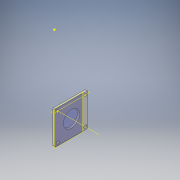
# Autodesk Inventor part: 30_Adapterplate_Eyepiece
Saved by Autodesk Inventor 2019 (Build 230136000, 136)
## iProperties
Created: 2018-06-14
Part Number: 30_Adapterplate_Eyepiece
Material: Generisch
Document SubType Name: Modeling
Designer: diederichbenedict
Density: 1 g/cm^3
Appearance: Vorgabe
Author: diederichbenedict
Autodesk Inventor part; units mm, degrees
ref_plane "YZ Plane" through (0, 0, 0) normal (1, 0, 0) x (0, 1, 0)
ref_plane "XZ Plane" through (0, 0, 0) normal (0, 1, 0) x (-1, 0, 0)
ref_plane "XY Plane" through (0, 0, 0) normal (0, 0, 1) x (1, 0, 0)
ref_plane "Arbeitsebene1" through (0, 0, -149.8) normal (-1, 0, 0) x (0, 0, 1)
sketch "Skizze1" plane through (0, 0, -149.8) normal (-1, 0, 0) x (0, 0, 1)
  circle A0 centre (44.9, 5) radius 1.5 construction
  circle A1 centre (4.9, 5) radius 1.5 construction
  circle A2 centre (4.9, 45) radius 1.6 construction
  circle A3 centre (44.9, 45) radius 1.6 construction
  line L0 (39.5269, 16.1776) -> (39.5269, 39.7) construction
  line L1 (16.0815, 10.3) -> (33.7185, 10.3) construction
  line L2 (10.2731, 16.1776) -> (10.2731, 39.7) construction
  circle A4 centre (24.9, 24.9269) radius 14.6269 construction
  line L3 (2, 49.8269) -> (47.8, 49.8269)
  line L4 (49.8, 47.8269) -> (49.8, 2.0269)
  line L5 (47.8, 0.0269) -> (2, 0.0269)
  line L6 (0, 2.0269) -> (0, 47.8269)
  line L7 (0, 49.8269) -> (49.8, 0.0269) construction
  line L8 (49.8, 49.8269) -> (0, 0.0269) construction
  arc A5 (47.8, 0.0269) -> (49.8, 2.0269) centre (47.8, 2.0269) ccw
  arc A6 (0, 2.0269) -> (2, 0.0269) centre (2, 2.0269) ccw
  arc A7 (2, 49.8269) -> (0, 47.8269) centre (2, 47.8269) ccw
  arc A8 (49.8, 47.8269) -> (47.8, 49.8269) centre (47.8, 47.8269) ccw
  line L9 (2, 1.0269) -> (47.8, 1.0269)
  arc A9 (47.8, 1.0269) -> (48.8, 2.0269) centre (47.8, 2.0269) ccw
  line L10 (48.8, 2.0269) -> (48.8, 47.8269)
  arc A10 (48.8, 47.8269) -> (47.8, 48.8269) centre (47.8, 47.8269) ccw
  line L11 (47.8, 48.8269) -> (2, 48.8269)
  arc A11 (2, 48.8269) -> (1, 47.8269) centre (2, 47.8269) ccw
  line L12 (1, 47.8269) -> (1, 2.0269)
  arc A12 (1, 2.0269) -> (2, 1.0269) centre (2, 2.0269) ccw
  point P0 (149.8, 0)
extrude "Extrusion1" add sketch "Skizze1" along normal blind 3 contours A12 L12 A11 L11 A10 L10 A9 L9
ref_plane "Arbeitsebene2" through (0, 5, -104.9) normal (0, 0, 1) x (1, 0, 0)
sketch "Skizze2" plane through (0, 5, -104.9) normal (0, 0, 1) x (1, 0, 0)
  line L0 (0, 5.3) -> (7, 5.3) projected
  line L1 (0, 8.3139) -> (7.3731, 8.3139)
  line L2 (0, -2.9731) -> (0, 42.8269) projected
  line L3 (0, 6.807) -> (-3, 6.807)
  line L4 (-3, -2.9731) -> (-3, 42.8269) projected
  circle A0 centre (-1.5, 6.807) radius 2.6
  line L5 (1.1, 6.807) -> (-4.1, 6.807)
  line L6 (0, 1.6861) -> (7.3731, 1.6861)
  line L7 (2.4, -2.5) -> (8, -2.5) projected
  line L8 (15, -1.5) -> (6.4, -1.5)
  line L9 (10.2731, 1.5) -> (6.4, 1.5)
  line L10 (0, -0.0077) -> (-3, -0.0077)
  circle A1 centre (-1.5, -0.0077) radius 2.6
  line L11 (1.1, -0.0077) -> (-4.1, -0.0077)
  line L12 (-7.92, 0) -> (18.82, 0) projected
  point P0 (0, -5)
  point P1 (0, 1.4993)
  dimension "d6" = 1.507
  dimension "d7" = 5.2
  dimension "d9" = 5.2
  constraints: 16 end point, 8 horizontal, 4 point on circle, 2 centre point, 2 midpoint, 2 point on line, 9 other
  measures "d6" distance between parallel lines of L0 L3
  measures "d7" diameter of A0
  measures "d9" diameter of A1
revolve "Umdrehung2" cut sketch "Skizze2" angle 360 about axis through (47.3, 5, -104.9) along (1, 0, 0) contours L11 A1 L2 | L2 A1 L4 L10 | L4 A1 L11
pattern_linear "Rechteckige Anordnung1" count 2 spacing 40 along (0, 1, 0) count 2 spacing 40 along (0, 0, -1) of "Umdrehung2"
sketch "Skizze3" plane through (0, 0, -149.8) normal (1, 0, 0) x (0, 0, -1)
  point P0 (-149.8, 0)
sketch "Skizze4" plane through (0, 0, -149.8) normal (1, 0, 0) x (0, 0, -1)
  circle A0 centre (-24.9, 25) radius 11.45
  circle A1 centre (-24.9, 25) radius 11.75
  point P0 (-149.8, 0)
  dimension "d18" = 0.3
  constraints: 2 centre point, 2 other
  measures "d18" radial gap between concentric circles of A0 A1
extrude "Extrusion2" cut sketch "Skizze4" against normal blind 10 contours A0 | A1
